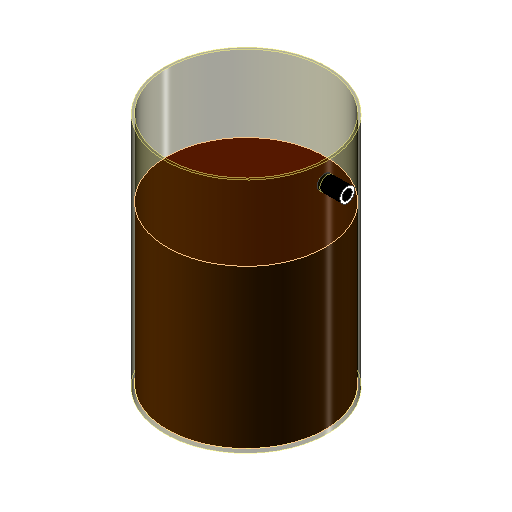
# Autodesk Inventor part: Cylinderical Container for AC3D Logo
Saved by Autodesk Inventor 2026.1 (Build 301233020, 233B)
## iProperties
Created: 2024-11-19
Part Number: Cylinderical Container for AC3D Logo
Material: Generic
Document SubType Name: Modeling
Designer: e3d
Density: 1 g/cm^3
Appearance: Default
Author: e3d
Autodesk Inventor part; units mm, degrees
ref_plane "YZ Plane" through (0, 0, 0) normal (1, 0, 0) x (0, 1, 0)
ref_plane "XZ Plane" through (0, 0, 0) normal (0, 1, 0) x (-1, 0, 0)
sketch "Sketch1" plane through (0, 0, 0) normal (0, 0, 1) x (1, 0, 0)
  line L0 (-41.91, 0) -> (251.46, 0) construction
  line L1 (0, -91.44) -> (0, 548.64) construction
  line L2 (203.2, 609.6) -> (209.55, 609.6)
  line L3 (209.55, 609.6) -> (209.55, 0)
  line L4 (209.55, 0) -> (203.2, 0)
  line L5 (203.2, 0) -> (203.2, 609.6)
  line L6 (203.2, 0) -> (0, 0)
  line L7 (0, 0) -> (0, 6.35)
  line L8 (0, 6.35) -> (203.2, 6.35)
  line L9 (203.2, 6.35) -> (203.2, 0)
  line L10 (203.2, 6.35) -> (0, 6.35)
  line L11 (0, 6.35) -> (0, 412.75)
  line L12 (0, 412.75) -> (203.2, 412.75)
  line L13 (203.2, 412.75) -> (203.2, 6.35)
  line L14 (0, 558.8) -> (260.35, 558.8) construction
  point P0 (203.2, 6.35)
  dimension "d0" = 203.2
  dimension "d1" = 609.6
  dimension "d2" = 6.35
  dimension "d3" = 406.4
  dimension "d6" = 50.8
  dimension "d7" = 50.8
  constraints: 26 end point, 6 parallel, 5 perpendicular, 4 point on line, 3 horizontal
  measures "d0" distance of L11.end L12.end
  measures "d1" distance of L2.end L3.end
  measures "d2" distance of L2.start L2.end
  measures "d3" distance of L12.end L8.end
  measures "d6" distance between parallel lines of L2 L14
  measures "d7" distance from line of L3 L14.end
revolve "Revolution1" add sketch "Sketch1" angle 360 about axis through (0, 6.35, 0) along (0, 1, 0) contours L5 L8 L11 L12
revolve "Revolution2" add sketch "Sketch1" angle 360 about axis through (0, -10, 0) along (0, 1, 0) separate body contours L2 L3 L4 L5 | L5 L6 L7 L8
ref_plane "Work Plane1 - Nozzle End" through (260.35, 558.8, 0) normal (1, 0, 0) x (0, 1, 0)
sketch "Sketch2" plane through (260.35, 558.8, 0) normal (1, 0, 0) x (0, 1, 0)
  circle A0 centre (0, 0) radius 12.7
  circle A1 centre (0, 0) radius 19.05
  dimension "d8" = 25.4
  dimension "d9" = 6.35
  constraints: 2 centre point, 1 coincident
  measures "d8" diameter of A0
  measures "d9" radial gap between concentric circles of A0 A1
extrude "Extrusion1 - Inlet Hole" cut sketch "Sketch2" against normal up to surface contours A0 | A1 round surface about axis through (0, 307.975, 0) along (0, 1, 0) radius 203.2 far side no bodies 2
extrude "Extrusion2" add sketch "Sketch2" against normal up to surface separate body round surface about axis through (0, 307.975, 0) along (0, 1, 0) radius 203.2 far side no
equation "\"d0\" = 0.5 * BaseDia"
equation "\"d1\" = TankHeight"
equation "\"d2\" = TankThickness"
equation "\"d3\" = LiquidDepth"
equation "\"d7\" = InletProjection"
equation "\"BaseDia\" = 406.4"
equation "\"TankHeight\" = 609.6"
equation "\"InletId\" = 21.336"
equation "\"InletThickness\" = 2.7686"
equation "\"LiquidDepth\" = 406.4"
equation "\"TankThickness\" = 6.35"
equation "\"InletProjection\" = 50.8"
